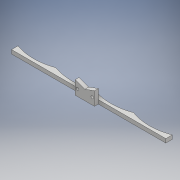
# Autodesk Inventor part: Biter
Saved by Autodesk Inventor 2018 (Build 220112000, 112)
## iProperties
Created: 2019-04-05
Part Number: Biter
Material: Типовые
Document SubType Name: Modeling
Designer: cosko
Density: 1 g/cm^3
Appearance: По умолчанию
Author: cosko
Autodesk Inventor part; units mm, degrees
ref_plane "YZ Plane" through (0, 0, 0) normal (1, 0, 0) x (0, 1, 0)
ref_plane "XZ Plane" through (0, 0, 0) normal (0, 1, 0) x (-1, 0, 0)
ref_plane "XY Plane" through (0, 0, 0) normal (0, 0, 1) x (1, 0, 0)
sketch "Эскиз2" plane through (0, 0, 0) normal (0, 0, 1) x (1, 0, 0)
  line L0 (-120, -5) -> (120, -5)
  line L1 (120, -5) -> (120, 5)
  line L2 (120, 5) -> (-120, 5)
  line L3 (-120, 5) -> (-120, -5)
  line L4 (-120, -5) -> (120, 5) construction
  line L5 (120, -5) -> (-120, 5) construction
  line L6 (-120, 5) -> (0, 5) construction
  line L7 (-61.2969, 5) -> (-61.2969, -5) construction
  line L8 (0, 5) -> (120, 5) construction
  line L9 (60, 5) -> (60, -5) construction
  arc A0 (-120, 5) -> (-61.2969, 5) centre (-90.6485, 86.3267) ccw
  arc A1 (-61.2969, 5) -> (0, 5) centre (-30.6485, 91.8022) ccw
  arc A2 (0, 5) -> (60, 5) centre (30, 85.0749) ccw
  arc A3 (60, 5) -> (120, 5) centre (90, 84.432) ccw
  point P0 (0, 0)
  dimension "d5" = 240
  dimension "d6" = 10
  constraints: 20 end point, 8 point on circle, 4 centre point, 4 midpoint, 4 perpendicular, 3 point on line, 2 parallel, 1 collinear, 1 horizontal
  measures "d5" distance of L2.end L1.end
  measures "d6" distance of L1.end L0.end
extrude "Выдавливание2" add sketch "Эскиз2" along normal blind 6 contours L3 A0 A1 A2 A3 L1 L0
sketch "Эскиз3" plane through (0, 0, 6) normal (0, 0, 1) x (1, 0, 0)
  line L0 (-120, -5) -> (120, -5) construction
  line L1 (0, -5) -> (15, -5) construction
  line L2 (15, -5) -> (-15, -5) construction
  line L3 (-15, -5) -> (15, -5)
  line L4 (15, -5) -> (15, -11)
  line L5 (15, -11) -> (-15, -11)
  line L6 (-15, -11) -> (-15, -5)
  point P0 (0, 0)
  dimension "d9" = 15
  dimension "d10" = 30
  dimension "d11" = 6
  constraints: 12 end point, 2 parallel, 2 point on line, 1 horizontal, 1 midpoint, 1 perpendicular
  measures "d9" distance of L1.start L1.end
  measures "d10" distance of L1.end L2.end
  measures "d11" distance of L3.end L4.end
extrude "Выдавливание3" add sketch "Эскиз3" along normal blind 15 and the other way blind 6
sketch "Эскиз4" plane through (-15, -11, 21) normal (0, -1, 0) x (1, 0, 0)
  line L0 (30, 0) -> (30, -21) projected
  line L1 (0, 0) -> (30, 0) projected
  line L2 (0, 0) -> (0, -21) projected
  line L3 (30, -21) -> (0, -21) projected
  line L4 (30, 0) -> (0, 0) construction
  line L5 (15, -21) -> (15, -15) construction
  line L6 (15, 0) -> (15, -21) construction
  line L7 (15, -10.5) -> (3.5, -10.5) construction
  line L8 (3.5, -10.5) -> (26.5, -10.5) construction
  circle A0 centre (3.5, -10.5) radius 2
  circle A1 centre (26.5, -10.5) radius 2
  line L9 (0, 0) -> (15, -5.4596)
  line L10 (0, 0) -> (15.9627, 0) construction
  line L11 (15, -5.4596) -> (30, 0)
  dimension "d16" = 11.5
  dimension "d17" = 23
  dimension "d18" = 4
  dimension "d19" = 4
  dimension "d22" = 20
  constraints: 12 end point, 2 centre point, 2 coincident, 2 horizontal, 2 midpoint, 2 point on line, 1 collinear, 1 equal length
  measures "d16" distance of L7.start L7.end
  measures "d17" distance of L7.end L8.end
  measures "d18" diameter of A0
  measures "d19" diameter of A1
  measures "d22" angle of L9 L10
extrude "Выдавливание4" cut sketch "Эскиз4" against normal blind 15 contours L11 L9 L1 | A0 | A1
